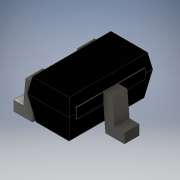
# Autodesk Inventor part: SOT523
Saved by Autodesk Inventor 2016 (Build 200138000, 138)
## iProperties
Created: 2016-09-07
Part Number: SOT523
Material: Generic
Document SubType Name: Modeling
Designer: jfixelle
Density: 1 g/cm^3
Appearance: Black
Author: jfixelle
Autodesk Inventor part; units mm, degrees
ref_plane "YZ Plane" through (0, 0, 0) normal (1, 0, 0) x (0, 1, 0)
ref_plane "XZ Plane" through (0, 0, 0) normal (0, 1, 0) x (-1, 0, 0)
ref_plane "XY Plane" through (0, 0, 0) normal (0, 0, 1) x (1, 0, 0)
sketch "Sketch1" plane through (0, 0, 0) normal (0, 1, 0) x (-1, 0, 0)
  line L0 (0.425, 0.85) -> (-0.425, 0.85)
  line L1 (-0.425, 0.85) -> (-0.425, -0.85)
  line L2 (-0.425, -0.85) -> (0.425, -0.85)
  line L3 (0.425, -0.85) -> (0.425, 0.85)
  point P0 (0, 0)
  dimension "d0" = 1.7
  dimension "d1" = 0.85
  dimension "d2" = 0.85
  dimension "d3" = 0.425
  constraints: 8 end point, 2 parallel, 1 horizontal, 1 perpendicular
  measures "d0" distance of L2.end L0.start
  measures "d1" distance from line of point (0, 0) L2
  measures "d2" distance of L1.end L2.end
  measures "d3" distance from line of point (0, 0) L3
extrude "Extrusion1" add sketch "Sketch1" along normal blind 0.8
chamfer "Chamfer1" distance 0.5 angle 10 1 edges at (-0.425, 0, 0) measured on face at (-0.425, 0.2667, -0.2833)
chamfer "Chamfer2" distance 0.5 angle 10 1 edges at (0.0441, 0, 0.85) measured on face at (0.1417, 0.4333, 0.85)
chamfer "Chamfer3" distance 0.5 angle 10 1 edges at (0.425, 0, -0.0441) measured on face at (0.425, 0.4333, -0.2833)
chamfer "Chamfer4" distance 0.5 angle 10 1 edges at (0, 0, -0.85) measured on face at (-0.1123, 0.3333, -0.85)
chamfer "Chamfer5" distance 0.3 angle 10 1 edges at (0.425, 0.8, 0) measured on face at (0.425, 0.7, -0.2833)
chamfer "Chamfer6" distance 0.3 angle 10 1 edges at (-0.0264, 0.8, -0.85) measured on face at (0.1241, 0.6, -0.85)
chamfer "Chamfer7" distance 0.3 angle 10 1 edges at (-0.425, 0.8, 0.0264) measured on face at (-0.425, 0.6, -0.2657)
chamfer "Chamfer8" distance 0.3 angle 10 1 edges at (0, 0.8, 0.85) measured on face at (-0.1241, 0.6001, 0.85)
sketch "Sketch2" plane through (0, 0, 0) normal (0, 0, 1) x (1, 0, 0)
  line L0 (0.232953, 0.6) -> (0.232953, 0.4)
  line L1 (0.232953, 0.4) -> (0.423178, 0.4)
  line L2 (0.423178, 0.4) -> (0.466922, -0.1)
  line L3 (0.466922, -0.1) -> (0.85, -0.1)
  line L4 (0.85, -0.1) -> (0.85, 0.1)
  line L5 (0.85, 0.1) -> (0.650188, 0.1)
  line L6 (0.650188, 0.1) -> (0.606444, 0.6)
  line L7 (0.606444, 0.6) -> (0.232953, 0.6)
  line L8 (0.425, 0.5) -> (-0.425, 0.5)
  line L9 (0, 0) -> (0, -0.071108)
  line L10 (-0.336837, 0) -> (0.336837, 0)
  dimension "d30" = 0.2
  dimension "d31" = 0.2
  dimension "d32" = 0.1
  dimension "d33" = 0.85
  dimension "d34" = 0.2
  dimension "d35" = 0.1
  dimension "d36" = 85
  constraints: 18 end point, 3 parallel, 3 perpendicular, 2 vertical
  measures "d30" distance of L3.end L4.end
  measures "d31" distance of L0.start L0.end
  measures "d32" distance between parallel lines of L7 L8
  measures "d33" distance between parallel lines of L4 L9
  measures "d34" distance between parallel lines of L6 L2
  measures "d35" distance between parallel lines of L3 L10
  measures "d36" angle of L5 L6
extrude "Extrusion2" add sketch "Sketch2" along normal mid plane 1.4
mirror "Mirror1" about plane through (0, 0, 0) normal (1, 0, 0) of "Extrusion2"
sketch "Sketch3" plane through (0, 0.8, 0) normal (0, 1, 0) x (1, 0, 0)
  line L0 (-0.423178, 0.7) -> (-0.423178, -0.7)
  line L1 (-0.987789, -0.35) -> (-0.423178, -0.35)
  line L2 (-0.423178, -0.35) -> (-0.423178, 0.35)
  line L3 (-0.423178, 0.35) -> (-0.987789, 0.35)
  line L4 (-0.987789, 0.35) -> (-0.987789, -0.35)
  line L5 (0.423178, 0.7) -> (0.423178, -0.7)
  line L6 (0.996529, 0.832609) -> (0.423178, 0.832609)
  line L7 (0.423178, 0.832609) -> (0.423178, 0.15)
  line L8 (0.423178, 0.15) -> (0.996529, 0.15)
  line L9 (0.996529, 0.15) -> (0.996529, 0.832609)
  line L10 (0.425, -0.7) -> (0.425, -0.85)
  line L11 (1.085249, -0.15) -> (0.425, -0.15)
  line L12 (0.425, -0.15) -> (0.425, -0.723836)
  line L13 (0.425, -0.723836) -> (1.085249, -0.723836)
  line L14 (1.085249, -0.723836) -> (1.085249, -0.15)
  point P0 (0, 0)
  dimension "d39" = 0.3
  dimension "d40" = 0.15
  dimension "d41" = 0.7
  dimension "d42" = 0.35
  constraints: 24 end point, 6 parallel, 3 horizontal, 3 perpendicular, 3 point on line
  measures "d39" distance between parallel lines of L11 L8
  measures "d40" distance from line of point (0, 0) L8
  measures "d41" distance of L3.end L1.start
  measures "d42" distance from line of point (0, 0) L1
sketch "Sketch3 outline for Extrusion3" plane through (0, 0.8, 0) normal (0, 1, 0) x (1, 0, 0)
  line L0 (1.085249, -0.723836) -> (1.085249, -0.15)
  line L1 (0.425, -0.723836) -> (1.085249, -0.723836)
  line L2 (0.425, -0.15) -> (0.425, -0.723836)
  line L3 (1.085249, -0.15) -> (0.425, -0.15)
  line L4 (0.996529, 0.15) -> (0.996529, 0.832609)
  line L5 (0.423178, 0.15) -> (0.996529, 0.15)
  line L6 (0.423178, 0.832609) -> (0.423178, 0.15)
  line L7 (0.996529, 0.832609) -> (0.423178, 0.832609)
  line L8 (-0.987789, 0.35) -> (-0.987789, -0.35)
  line L9 (-0.423178, 0.35) -> (-0.987789, 0.35)
  line L10 (-0.423178, -0.35) -> (-0.423178, 0.35)
  line L11 (-0.987789, -0.35) -> (-0.423178, -0.35)
extrude "Extrusion3" cut sketch "Sketch3 outline for Extrusion3" against normal blind 1.4
body "Solid1"
